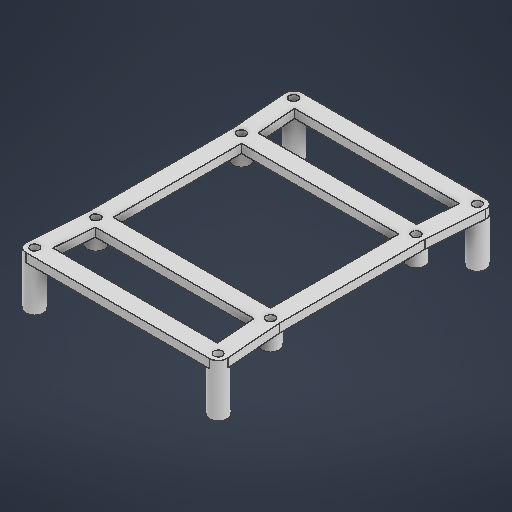
# Autodesk Inventor part: RP_mounting_cover
Saved by Autodesk Inventor 2026.1 (Build 301233000, 233)
## iProperties
Created: 2026-03-24
Part Number: RP_mounting_cover
Material: Generic
Document SubType Name: Modeling
Designer: emanuel
Density: 1 g/cm^3
Appearance: Default
Author: emanuel
Autodesk Inventor part; units mm, degrees
ref_plane "YZ Plane" through (0, 0, 0) normal (1, 0, 0) x (0, 1, 0)
ref_plane "XZ Plane" through (0, 0, 0) normal (0, 1, 0) x (-1, 0, 0)
ref_plane "XY Plane" through (0, 0, 0) normal (0, 0, 1) x (1, 0, 0)
sketch "Sketch1" plane through (0, 0, 0) normal (0, 1, 0) x (-1, 0, 0)
  line L0 (0, 0) -> (63, 0)
  line L1 (63, 0) -> (63, -89)
  line L2 (63, -89) -> (0, -89)
  line L3 (0, -89) -> (0, 0)
  circle A0 centre (0, 0) radius 1.5
  circle A1 centre (63, 0) radius 1.5
  circle A2 centre (0, -89) radius 1.5
  circle A3 centre (63, -89) radius 1.5
  circle A4 centre (0, 0) radius 3
  circle A5 centre (0, -89) radius 3
  circle A6 centre (63, -89) radius 3
  circle A7 centre (63, 0) radius 3
  dimension "d0" = 63
  dimension "d1" = 89
  dimension "d2" = 3
  dimension "d3" = 3
  dimension "d4" = 3
  dimension "d5" = 3
  dimension "d6" = 6
  dimension "d7" = 6
  dimension "d8" = 6
  dimension "d9" = 6
  constraints: 8 centre point, 8 coincident, 8 end point, 2 parallel, 1 horizontal, 1 perpendicular
  measures "d0" distance of L1.end L2.end
  measures "d1" distance of L0.end L1.end
  measures "d2" diameter of A0
  measures "d3" diameter of A1
  measures "d4" diameter of A2
  measures "d5" diameter of A3
  measures "d6" diameter of A4
  measures "d7" diameter of A5
  measures "d8" diameter of A6
  measures "d9" diameter of A7
extrude "Extrusion1" add sketch "Sketch1" along normal blind 15 contours A0 L3 A4 L0 | L0 A4 L3 A0 | A7 L1 A1 L0 | L0 A1 L1 A7 | A5 L2 A2 L3 | L3 A2 L2 A5 | A6 L2 A3 L1 | L1 A3 L2 A6
sketch "Sketch2" plane through (0, 15, 0) normal (0, 1, 0) x (1, 0, 0)
  circle A0 centre (0, 0) radius 1.5 projected
  circle A1 centre (-63, 89) radius 1.5 projected
  line L0 (0, 0) -> (-63, 0)
  line L1 (-63, 0) -> (-63, 89)
  line L2 (-63, 89) -> (0, 89)
  line L3 (0, 89) -> (0, 0)
  line L4 (-63, 44.5) -> (-31.5, 44.5)
  line L5 (-1.5, 19.5) -> (-61.5, 19.5)
  line L6 (-61.5, 19.5) -> (-61.5, 69.5)
  line L7 (-61.5, 69.5) -> (-1.5, 69.5)
  line L8 (-1.5, 69.5) -> (-1.5, 19.5)
  line L9 (-1.5, 19.5) -> (-61.5, 69.5) construction
  line L10 (-61.5, 19.5) -> (-1.5, 69.5) construction
  circle A2 centre (-61.5, 19.5) radius 1.5
  circle A3 centre (-1.5, 19.5) radius 1.5
  circle A4 centre (-1.5, 69.5) radius 1.5
  circle A5 centre (-61.5, 69.5) radius 1.5
  circle A6 centre (-61.5, 19.5) radius 3
  circle A7 centre (-61.5, 69.5) radius 3
  circle A8 centre (-1.5, 19.5) radius 3
  circle A9 centre (-1.5, 69.5) radius 3
  dimension "d12" = 60
  dimension "d13" = 50
  dimension "d14" = 3
  dimension "d15" = 3
  dimension "d16" = 3
  dimension "d17" = 3
  dimension "d18" = 6
  dimension "d19" = 6
  dimension "d20" = 6
  dimension "d21" = 6
  constraints: 22 end point, 8 centre point, 8 coincident, 4 parallel, 3 horizontal, 3 midpoint, 2 perpendicular
  measures "d12" distance of L6.end L7.end
  measures "d13" distance of L5.end L6.end
  measures "d14" diameter of A2
  measures "d15" diameter of A3
  measures "d16" diameter of A4
  measures "d17" diameter of A5
  measures "d18" diameter of A6
  measures "d19" diameter of A7
  measures "d20" diameter of A8
  measures "d21" diameter of A9
extrude "Extrusion2" add sketch "Sketch2" against normal blind 5 contours A8 L5 A3 L3 | L3 A8 | A3 L8 A8 L3 | A8 L8 A3 L5 | A6 L1 | L1 A2 L5 A6 | L5 A2 L6 A6 | L1 A6 L6 A2 | A9 L8 A4 L3 | L3 A9 | A9 L7 A4 L8 | A4 L7 A9 L3 | A7 L1 | L1 A5 L6 A7 | L6 A5 L7 A7 | L7 A5 L1 A7
sketch "Sketch3" plane through (-63, 15, 0) normal (0, 1, 0) x (1, 0, 0)
  circle A0 centre (0, 0) radius 1.5 projected
  circle A1 centre (1.5, 19.5) radius 1.5 projected
  line L0 (0, 0) -> (1.5, 19.5) construction
  line L1 (2.9912, -0.2301) -> (4.4912, 19.2699)
  line L2 (-1.4912, 19.7301) -> (-2.9912, 0.2301)
  arc A2 (-2.9912, 0.2301) -> (2.9912, -0.2301) centre (0, 0) ccw
  arc A3 (4.4912, 19.2699) -> (-1.4912, 19.7301) centre (1.5, 19.5) ccw
  circle A4 centre (1.5, 69.5) radius 1.5 projected
  line L3 (1.5, 19.5) -> (1.5, 69.5) construction
  line L4 (-1.5, 19.5) -> (-1.5, 69.5)
  line L5 (4.5, 69.5) -> (4.5, 19.5)
  arc A5 (-1.5, 19.5) -> (4.5, 19.5) centre (1.5, 19.5) ccw
  arc A6 (4.5, 69.5) -> (-1.5, 69.5) centre (1.5, 69.5) ccw
  circle A7 centre (0, 89) radius 1.5 projected
  line L6 (1.5, 69.5) -> (0, 89) construction
  line L7 (-1.4824, 69.2706) -> (-2.9824, 88.7706)
  line L8 (2.9824, 89.2294) -> (4.4824, 69.7294)
  arc A8 (-1.4824, 69.2706) -> (4.4824, 69.7294) centre (1.5, 69.5) ccw
  arc A9 (2.9824, 89.2294) -> (-2.9824, 88.7706) centre (0, 89) ccw
  circle A10 centre (63, 89) radius 1.5 projected
  line L9 (0, 89) -> (63, 89) construction
  line L10 (0, 86.0176) -> (63, 86.0176)
  line L11 (63, 91.9824) -> (0, 91.9824)
  arc A11 (0, 91.9824) -> (0, 86.0176) centre (0, 89) ccw
  arc A12 (63, 86.0176) -> (63, 91.9824) centre (63, 89) ccw
  circle A13 centre (61.5, 69.5) radius 1.5 projected
  line L12 (63, 89) -> (61.5, 69.5) construction
  line L13 (60.0176, 89.2294) -> (58.5176, 69.7294)
  line L14 (64.4824, 69.2706) -> (65.9824, 88.7706)
  arc A14 (65.9824, 88.7706) -> (60.0176, 89.2294) centre (63, 89) ccw
  arc A15 (58.5176, 69.7294) -> (64.4824, 69.2706) centre (61.5, 69.5) ccw
  circle A16 centre (61.5, 19.5) radius 1.5 projected
  line L15 (61.5, 69.5) -> (61.5, 19.5) construction
  line L16 (58.5, 69.5) -> (58.5, 19.5)
  line L17 (64.5, 19.5) -> (64.5, 69.5)
  arc A17 (64.5, 69.5) -> (58.5, 69.5) centre (61.5, 69.5) ccw
  arc A18 (58.5, 19.5) -> (64.5, 19.5) centre (61.5, 19.5) ccw
  line L18 (61.5, 19.5) -> (63, 0) construction
  line L19 (58.5176, 19.2706) -> (60.0176, -0.2294)
  line L20 (65.9824, 0.2294) -> (64.4824, 19.7294)
  arc A19 (64.4824, 19.7294) -> (58.5176, 19.2706) centre (61.5, 19.5) ccw
  arc A20 (60.0176, -0.2294) -> (65.9824, 0.2294) centre (63, 0) ccw
  line L21 (63, 0) -> (0, 0) construction
  line L22 (63, 3) -> (0, 3)
  line L23 (0, -3) -> (63, -3)
  arc A21 (63, -3) -> (63, 3) centre (63, 0) ccw
  arc A22 (0, 3) -> (0, -3) centre (0, 0) ccw
  line L24 (1.5, 19.5) -> (61.5, 19.5) construction
  line L25 (1.5, 16.5176) -> (61.5, 16.5176)
  line L26 (61.5, 22.4824) -> (1.5, 22.4824)
  arc A23 (1.5, 22.4824) -> (1.5, 16.5176) centre (1.5, 19.5) ccw
  arc A24 (61.5, 16.5176) -> (61.5, 22.4824) centre (61.5, 19.5) ccw
  line L27 (1.5, 69.5) -> (61.5, 69.5) construction
  line L28 (1.5, 72.4824) -> (61.5, 72.4824)
  line L29 (61.5, 66.5176) -> (1.5, 66.5176)
  arc A25 (1.5, 72.4824) -> (1.5, 66.5176) centre (1.5, 69.5) ccw
  arc A26 (61.5, 66.5176) -> (61.5, 72.4824) centre (61.5, 69.5) ccw
  circle A27 centre (63, 0) radius 1.5 projected
  circle A28 centre (63, 0) radius 1.5
  circle A29 centre (63, 89) radius 1.5
  circle A30 centre (0, 89) radius 1.5
  point P0 (0.75, 9.75)
  point P1 (1.5, 44.5)
  point P2 (0.75, 79.25)
  point P3 (31.5, 89)
  point P4 (62.25, 79.25)
  point P5 (61.5, 44.5)
  point P6 (62.25, 9.75)
  point P7 (31.5, 0)
  point P8 (31.5, 19.5)
  point P9 (31.5, 69.5)
  point P10 (0.2294, 91.9824)
  point P11 (-1.5, 69.5)
  point P12 (-1.5, 19.6152)
  point P13 (65.9648, 0.4582)
  point P14 (64.5, 19.5007)
  point P15 (62.7706, 91.9824)
  point P16 (58.7294, 16.5176)
  point P17 (59.7692, 3)
  point P18 (3.2396, 3)
  point P19 (4.2794, 16.5176)
  point P20 (58.5, 22.4824)
  point P21 (4.5, 22.4824)
  point P22 (4.5, 66.5176)
  point P23 (58.5, 66.5176)
  point P24 (3.2294, 86.0176)
  point P25 (59.7706, 86.0176)
  point P26 (58.7294, 72.4824)
  point P27 (4.2706, 72.4824)
  constraints: 80 end point, 40 point on circle, 40 tangent, 23 centre point, 12 parallel, 10 midpoint, 5 perpendicular, 3 coincident, 2 concentric, 1 vertical
extrude "Extrusion3" add sketch "Sketch3" along normal blind 3 contours A2 A22 L22 L1 | L1 L22 L19 A20 L20 A21 L23 A2 | L22 A22 L2 L4 A5 L25 L1 | L25 A5 L1 | L1 A3 L5 L26 L16 A18 L19 L25 | L22 A21 L20 A20 L19 | L19 L25 A18 L20 A21 L22 | A5 L25 A23 L26 A3 | A5 L4 L2 A3 L26 A23 L25 | L19 A18 L25 | L4 L7 A8 L29 L5 L26 A3 L2 | A3 L26 L5 | L19 A19 L26 A24 L25 A18 | A18 L16 L26 A19 L19 | L25 A24 L26 A19 L20 A18 | L7 A9 L11 A11 L10 L8 L28 A6 | A6 L28 A25 L29 A8 L7 | L20 A19 L26 L16 L29 A15 L14 L17 | L28 L8 A6 | A6 L8 A8 L29 A25 L28 | A17 L28 L13 L10 A12 L11 A14 L14 | L14 A15 L29 A26 L28 A17 | L29 A8 L8 A6 L5 | L5 A6 L8 L28 L13 A17 L16 L29 | L11 A14 L13 L10 L8 A9 | A9 L8 L10 A11 L11 | L28 A26 L29 A15 L13 A17 | A17 L13 L28 | L16 A17 L13 A15 L29 | L11 A12 L10 L13 A14
body "Solid1"
